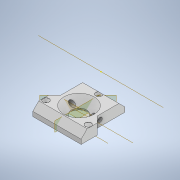
# Autodesk Inventor part: 20_Cube_Insert_Fibercombiner_FPC_filtermount_12.5mmRound_v3
Saved by Autodesk Inventor 2022 (Build 260153000, 153)
## iProperties
Created: 2021-12-04
Part Number: 20_Cube_Insert_Fibercombiner_FPC_filtermount_12.5mmRound_v3
Material: Generisch
Document SubType Name: Modeling
Designer: diederichbenedict
Density: 1 g/cm^3
Appearance: Vorgabe
Author: diederichbenedict
Autodesk Inventor part; units mm, degrees
ref_plane "YZ Plane" through (0, 0, 0) normal (1, 0, 0) x (0, 1, 0)
ref_plane "XZ Plane" through (0, 0, 0) normal (0, 1, 0) x (-1, 0, 0)
ref_plane "XY Plane" through (0, 0, 0) normal (0, 0, 1) x (1, 0, 0)
sketch "Skizze1" plane through (0, 0, 0) normal (0, 1, 0) x (-1, 0, 0)
  line L0 (0, 0) -> (-18, 0)
  line L1 (-18, 0) -> (-18, 28)
  line L2 (-18, 28) -> (0, 28)
  line L3 (0, 28) -> (0, 0)
  dimension "d0" = 18
  dimension "d1" = 28
  constraints: 8 end point, 2 parallel, 1 horizontal, 1 perpendicular
  measures "d0" distance of L1.end L2.end
  measures "d1" distance of L0.end L1.end
extrude "Extrusion1" add sketch "Skizze1" along normal blind 7
ref_plane "Arbeitsebene2" through (9, 0, 0) normal (-0.7071068, 0, -0.7071068) x (0, 1, 0)
ref_plane "Arbeitsebene1" through (9, 0, 0) normal (-1, 0, 0) x (0, 0, 1)
ref_plane "Arbeitsebene3" through (0, 0, 14) normal (0, 0, 1) x (1, 0, 0)
sketch "Skizze6" plane through (0, 0, 0) normal (-1, 0, 0) x (0, 0, 1)
  line L0 (0, 7) -> (28, 7) projected
  line L1 (0, 0) -> (0, 7) projected
  line L2 (0, 0) -> (28, 0) projected
  line L3 (28, 0) -> (28, 7) projected
  line L4 (0, 7) -> (-5, 7)
  line L5 (-5, 7) -> (-5, 0)
  line L6 (-5, 0) -> (0, 0)
  line L7 (0, 0) -> (0, 7)
  dimension "d24" = 5
  constraints: 8 end point, 2 parallel, 1 coincident, 1 horizontal, 1 perpendicular
  measures "d24" distance of L6.end L5.end
extrude "Extrusion6" add sketch "Skizze6" against normal up to surface (18 mm away) contours L1 L6 L5 L4
ref_plane "Arbeitsebene4" through (-15.85, 34.42605, 14.084853) normal (0, 0.7071068, -0.7071068) x (1, 0, 0)
sketch "Skizze7" plane through (-15.85, 34.42605, 14.084853) normal (0, 0.7071068, -0.7071068) x (1, 0, 0)
  point P0 (15.85, 34.302388)
sketch "Skizze8" plane through (0, 0, 0) normal (0, -1, 0) x (1, 0, 0)
  line L0 (0, 28) -> (18, 28) projected
  line L1 (18, 28) -> (18, -5) projected
  line L2 (0, -5) -> (0, 28) projected
  line L3 (0, -5) -> (-3, -5)
  line L4 (-3, -5) -> (-3, 28)
  line L5 (-3, 28) -> (0, 28)
  line L6 (0, 28) -> (0, -5)
  line L7 (18, 28) -> (18, -5) projected
  line L8 (18, 28) -> (21, 28)
  line L9 (21, 28) -> (21, -5)
  line L10 (21, -5) -> (18, -5)
  line L11 (18, -5) -> (18, 28)
  line L12 (0, -5) -> (0, 28) projected
  line L13 (0, -5) -> (18, -5) projected
  point P0 (0, 0)
  dimension "d27" = 3
  dimension "d28" = 3
  constraints: 16 end point, 4 parallel, 2 horizontal, 2 perpendicular, 1 point on line
  measures "d27" distance of L4.end L5.end
  measures "d28" distance of L9.end L10.end
extrude "Extrusion7" add sketch "Skizze8" against normal blind 7 contours L2 L3 L4 L5 | L8 L9 L10 L1
ref_plane "Arbeitsebene5" through (21, -5.727922, 12.727922) normal (0, 0.7071068, -0.7071068) x (-1, 0, 0)
sketch "Skizze10" plane through (-3, 0, -5) normal (-1, 0, 0) x (0, 0, 1)
  line L0 (0, 7) -> (33, 7)
  line L1 (0, 0) -> (0, 7)
  line L2 (33, 0) -> (0, 0)
  line L3 (33, 0) -> (33, 7)
  circle A0 centre (16.5, 3.919305) radius 1.45
  point P0 (5, 0)
  dimension "d38" = 2.9
  constraints: 1 centre point
  measures "d38" diameter of A0
extrude "Extrusion9" cut sketch "Skizze10" against normal through all contours A0
ref_plane "Arbeitsebene6" through (21, -1.485281, 8.485281) normal (0, 0.7071068, -0.7071068) x (-1, 0, 0)
sketch "Skizze14" plane through (21, 0, -5) normal (0, 0, -1) x (-1, 0, 0)
  line L0 (24, 0) -> (0, 0)
  line L1 (3.75, 1.4) -> (20.25, 1.4)
  circle A0 centre (17.510731, 1.4) radius 0.9
  circle A1 centre (7.176394, 1.4) radius 1.009656
  point P0 (21, 0)
  dimension "d55" = 1.8
  constraints: 2 centre point, 1 point on line
  measures "d55" diameter of A0
hole "Bohrung3" at (3.489269, 1.4, -5) at (13.823606, 1.4, -5) direction (0, 0, 1) diameter 1.8 depth 10 tip angle 118 counterbore diameter 4 counterbore depth 4
sketch "Skizze15" plane through (21, 0, 28) normal (1, 0, 0) x (0, 0, -1)
  circle A0 centre (16.5, 3.919305) radius 1.45
  line L0 (0, 7) -> (33, 7)
  line L1 (0, 0) -> (0, 7)
  line L2 (33, 0) -> (0, 0)
  line L3 (33, 0) -> (33, 7)
  line L4 (25.25, 7) -> (5, 7)
  line L5 (10.609557, 7) -> (10.609557, 0)
  point P0 (28, 0)
  constraints: 2 end point, 2 point on line, 1 perpendicular
extrude "Extrusion10" add sketch "Skizze15" along normal blind 4 contours L0 L5 L2 L1
sketch "Skizze16" plane through (-3, 0, -5) normal (-1, 0, 0) x (0, 0, 1)
  line L0 (33, 7) -> (33, 0)
  line L1 (33, 0) -> (22.390443, 0)
  line L2 (22.390443, 0) -> (22.390443, 7)
  line L3 (22.390443, 7) -> (33, 7)
  point P0 (5, 0)
extrude "Extrusion11" add sketch "Skizze16" along normal blind 4
sketch "Skizze13" plane through (21, 7, 8.485281) normal (0, 1, 0) x (-1, 0, 0)
  circle A0 centre (-2, 12.771292) radius 2.45
  circle A1 centre (26, 12.771292) radius 2.45
  circle A2 centre (12, -8.228708) radius 2.75
  point P0 (21, -4.949747)
  point P1 (12, -10.228708)
hole "Bohrung2" at (23, 7, 21.256574) at (-5, 7, 21.256574) at (9, 7, 0.256574) direction (0, -1, 0) diameter 4 depth 0.1 tip angle 118
chamfer "Fase3" distance 4 angle 45 4 edges at (21, 3.5, 17.3904) (-3, 3.5, 17.3904) (9, 7, 28) (9, 7, -5)
sketch "Sketch17" plane through (0, 0, 0) normal (0, -1, 0) x (1, 0, 0)
  line L0 (2.060983, -5) -> (2.060983, -1)
  line L1 (2.060983, -1) -> (4.917554, -1)
  line L2 (4.917554, -1) -> (4.917554, -5)
  line L3 (4.917554, -5) -> (12.39532, -5)
  line L4 (12.39532, -5) -> (12.39532, -1)
  line L5 (12.39532, -1) -> (15.251891, -1)
  line L6 (15.251891, -1) -> (15.251891, -5)
  line L7 (15.251891, -5) -> (21, -5)
  line L8 (21, -5) -> (21, 13.390443)
  line L9 (25, 17.390443) -> (21, 13.390443)
  line L10 (25, 28) -> (25, 17.390443)
  line L11 (-7, 28) -> (25, 28)
  line L12 (-7, 17.390443) -> (-7, 28)
  line L13 (-3, 13.390443) -> (-7, 17.390443)
  line L14 (-3, 13.390443) -> (-3, -5)
  line L15 (-3, -5) -> (2.060983, -5)
  circle A0 centre (9, 13.390443) radius 6.35
  point P0 (0, 0)
  dimension "d70" = 12.7
  constraints: 1 centre point
  measures "d70" diameter of A0
extrude "Extrusion12" cut sketch "Sketch17" against normal blind 2 contours A0
sketch "Sketch18" plane through (0, 7, 0) normal (0, 1, 0) x (1, 0, 0)
  circle A0 centre (9, -13.390443) radius 6.35
  circle A1 centre (9, -13.390443) radius 10
  point P0 (0, 0)
  dimension "d73" = 20
  constraints: 1 centre point, 1 coincident
  measures "d73" diameter of A1
sketch "Sketch18 outline for Extrusion13" plane through (0, 7, 0) normal (0, 1, 0) x (1, 0, 0)
  circle A0 centre (9, -13.390443) radius 10
extrude "Extrusion13" cut sketch "Sketch18 outline for Extrusion13" against normal up to surface (5 mm away) draft -45
